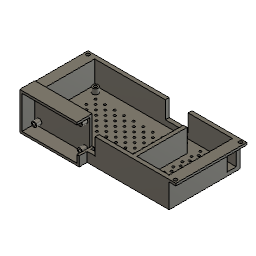
PCB+Case (Autodesk Fusion 360 design; units mm, degrees)
Autodesk Fusion 360 part; units mm, degrees
sketch "Sketch1" plane through (0, 0, 0) normal (0, 1, 0) x (1, 0, 0)
  line L0 (-72.5, 44.98) -> (120.5, 44.98)
  line L1 (120.5, 44.98) -> (120.5, -49.32)
  line L2 (120.5, -49.32) -> (-72.5, -49.32)
  line L3 (-72.5, -49.32) -> (-72.5, 44.98)
  line L4 (-67.5, 39.83) -> (67.5, 39.83)
  line L5 (67.5, 39.83) -> (67.5, -39.83)
  line L6 (67.5, -39.83) -> (-67.5, -39.83)
  line L7 (-67.5, -39.83) -> (-67.5, 39.83)
  circle A0 centre (-58.42, 31.75) radius 1.9
  circle A1 centre (-58.42, -31.75) radius 1.9
  circle A2 centre (58.42, 31.75) radius 1.9
  circle A3 centre (58.42, -31.75) radius 1.9
  circle A4 centre (-58.42, 31.75) radius 3.9
  circle A5 centre (58.42, 31.75) radius 3.9
  circle A6 centre (58.42, -31.75) radius 3.9
  circle A7 centre (-58.42, -31.75) radius 3.9
  line L8 (72.5, 39.83) -> (115.5, 39.83)
  line L9 (115.5, 39.83) -> (115.5, -44.17)
  line L10 (115.5, -44.17) -> (72.5, -44.17)
  line L11 (72.5, -44.17) -> (72.5, 39.83)
  line L12 (67.5, 39.83) -> (72.5, 39.83) construction
  dimension "d1" = 135
  dimension "d2" = 67.5
  dimension "d3" = 79.66
  dimension "d4" = 39.83
  dimension "d5" = 5.15
  dimension "d8" = 5
  dimension "d9" = 58.42
  dimension "d10" = 58.42
  dimension "d11" = 58.42
  dimension "d12" = 58.42
  dimension "d13" = 31.75
  dimension "d14" = 31.75
  dimension "d15" = 31.75
  dimension "d16" = 31.75
  dimension "d17" = 3.8
  dimension "d18" = 3.8
  dimension "d19" = 3.8
  dimension "d20" = 3.8
  dimension "d21" = 7.8
  dimension "d22" = 7.8
  dimension "d23" = 7.8
  dimension "d24" = 7.8
  dimension "d111" = 43
  dimension "d112" = 84
  dimension "d113" = 5.15
  dimension "d114" = 5
  dimension "d115" = 5
  constraint horizontal L0
  constraint vertical L1
  constraint horizontal L2
  constraint vertical L3
  constraint horizontal L4
  constraint vertical L5
  constraint horizontal L6
  constraint vertical L7
  constraint concentric A0 A4
  constraint concentric A2 A5
  constraint concentric A3 A6
  constraint concentric A1 A7
  constraint horizontal L8
  constraint vertical L9
  constraint horizontal L10
  constraint vertical L11
  constraint horizontal L12
  measures "d1" distance of L4.start L4.end
  measures "d2" distance of origin L5
  measures "d3" distance of L4.start L6.end
  measures "d4" distance of origin L4
  measures "d5" distance of L0 L4
  measures "d8" distance of L3 L7
  measures "d9" horizontal distance of origin A0.centre
  measures "d10" horizontal distance of origin A2.centre
  measures "d11" horizontal distance of origin A1.centre
  measures "d12" horizontal distance of origin A3.centre
  measures "d13" vertical distance of origin A0.centre
  measures "d14" vertical distance of origin A2.centre
  measures "d15" vertical distance of origin A1.centre
  measures "d16" vertical distance of origin A3.centre
  measures "d17" diameter of A0
  measures "d18" diameter of A2
  measures "d19" diameter of A1
  measures "d20" diameter of A3
  measures "d21" diameter of A4
  measures "d22" diameter of A5
  measures "d23" diameter of A7
  measures "d24" diameter of A6
  measures "d111" distance of L8.start L8.end
  measures "d112" distance of L8.end L9.end
  measures "d113" distance of L2 L10
  measures "d114" distance of L1 L9
  measures "d115" distance of L5 L11
extrude "Extrude1" add sketch "Sketch1" along normal blind 5 contours L4 L5 L6 L7 | A4 | A5 | A6 | A7 | L8 L9 L10 L11 makes body 1 at (-18.887, 0, 10.2448) makes body 2 at (86.8333, 0, 16.17)
extrude "Extrude3" add sketch "Sketch1" along normal blind 35 contours L0 L1 L2 L3 bodies 1 2
extrude "Extrude15" add sketch "Sketch1" along normal blind 5 contours A0 | A1 | A2 | A3 bodies 1
extrude "Extrude16" add sketch "Sketch1" along normal blind 12 contours A4 | A5 | A6 | A7 bodies 1
sketch "Sketch11" plane through (0, 35, 0) normal (0, 1, 0) x (-1, 0, 0)
  line L0 (-67.5, 39.83) -> (67.5, 39.83)
  line L1 (67.5, 39.83) -> (67.5, -39.83)
  line L2 (67.5, -39.83) -> (-67.5, -39.83)
  line L3 (-67.5, -39.83) -> (-67.5, 39.83)
  line L4 (-115.5, 44.17) -> (-72.5, 44.17)
  line L5 (-72.5, 44.17) -> (-72.5, -39.83)
  line L6 (-72.5, -39.83) -> (-115.5, -39.83)
  line L7 (-115.5, -39.83) -> (-115.5, 44.17)
  line L8 (72.5, 49.32) -> (-120.5, 49.32)
  line L9 (-120.5, 49.32) -> (-120.5, -44.98)
  line L10 (-120.5, -44.98) -> (72.5, -44.98)
  line L11 (72.5, -44.98) -> (72.5, 49.32)
  line L12 (72.5, 49.32) -> (-67.5, 49.32)
  line L13 (-67.5, 49.32) -> (-67.5, 44.83)
  line L14 (-67.5, 44.83) -> (72.5, 44.83)
  line L15 (72.5, 44.83) -> (72.5, 49.32)
  line L16 (-67.5, 44.83) -> (-67.5, 39.83)
  dimension "d117" = 5
  constraint horizontal L12
  constraint vertical L13
  constraint horizontal L14
  constraint vertical L15
  constraint coincident L8.start L11.end
  constraint coincident L0.start L3.end
  constraint vertical L16
  measures "d117" distance of L0 L14
extrude "Extrude11" cut sketch "Sketch11" against normal up to surface (35 mm away) contours L8 L11 L12 L13 L14 L15 bodies 1
sketch "Sketch2" plane through (0, 35, 0) normal (0, 1, 0) x (-1, 0, 0)
  line L0 (-67.5, 39.83) -> (67.5, 39.83)
  line L1 (67.5, 39.83) -> (67.5, -39.83)
  line L2 (67.5, -39.83) -> (-67.5, -39.83)
  line L3 (-67.5, -39.83) -> (-67.5, 39.83)
  line L4 (-67.5, 49.32) -> (-120.5, 49.32)
  line L5 (-120.5, 49.32) -> (-120.5, -44.98)
  line L6 (-120.5, -44.98) -> (72.5, -44.98)
  line L7 (72.5, -44.98) -> (72.5, 44.83)
  line L8 (81.5, -44.98) -> (-129.5, -44.98)
  line L9 (-129.5, -44.98) -> (-129.5, 49.32)
  line L10 (81.5, 44.83) -> (81.5, -44.98)
  circle A0 centre (77, 40.33) radius 2.25
  circle A1 centre (77, -40.48) radius 2.25
  circle A2 centre (-125, -40.98) radius 2.25
  circle A3 centre (-125, 45.32) radius 2.25
  line L11 (-115.5, 44.17) -> (-72.5, 44.17)
  line L12 (-72.5, 44.17) -> (-72.5, -39.83)
  line L13 (-72.5, -39.83) -> (-115.5, -39.83)
  line L14 (-115.5, -39.83) -> (-115.5, 44.17)
  line L15 (-67.5, 44.83) -> (-67.5, 49.32)
  line L16 (72.5, 44.83) -> (-67.5, 44.83)
  line L17 (-129.5, 49.32) -> (-120.5, 49.32)
  line L18 (72.5, 44.83) -> (81.5, 44.83)
  point P0 (-24, -44.98)
  dimension "d33" = 9
  dimension "d39" = 4.5
  dimension "d40" = 4.5
  dimension "d41" = 4.5
  dimension "d42" = 4.5
  dimension "d43" = 4
  dimension "d44" = 4.5
  dimension "d46" = 4.5
  dimension "d47" = 4.5
  dimension "d48" = 4.5
  dimension "d50" = 4.5
  dimension "d116" = 9
  dimension "d121" = 4
  dimension "d122" = 4.5
  constraint horizontal L8
  constraint vertical L9
  constraint vertical L10
  constraint midpoint L6 P0
  constraint coincident L8 P0
  constraint coincident L4.end L5.start
  constraint perpendicular L5 L17
  constraint coincident L7.end L16.start
  constraint horizontal L18
  measures "d33" distance of L7 L10
  measures "d39" distance of L10 A1.centre
  measures "d40" distance of L8 A1.centre
  measures "d41" diameter of A1
  measures "d42" distance of L9 A2.centre
  measures "d43" distance of L8 A2.centre
  measures "d44" diameter of A2
  measures "d46" distance of L10 A0.centre
  measures "d47" diameter of A0
  measures "d48" distance of L9 A3.centre
  measures "d50" diameter of A3
  measures "d116" distance of L5 L9
  measures "d121" distance of A3.centre L17
  measures "d122" distance of A0.centre L18
extrude "Extrude4" add sketch "Sketch2" against normal blind 3 contours L5 L8 L9 L17 | L7 L8 L10 L18 bodies 1
sketch "Sketch7" plane through (0, 35, 0) normal (0, 1, 0) x (-1, 0, 0)
  line L0 (81.5, -44.98) -> (81.5, 44.83)
  line L1 (-67.5, 49.32) -> (-129.5, 49.32)
  circle A0 centre (77, 40.33) radius 2.25
  line L2 (67.5, 39.83) -> (-11.62, 39.83)
  line L3 (67.5, 59.83) -> (67.5, 39.83)
  line L4 (-11.62, 39.83) -> (-11.62, 59.83)
  line L5 (67.5, 59.83) -> (-11.62, 59.83)
  line L6 (-129.5, -44.98) -> (81.5, -44.98)
  circle A1 centre (77, -40.48) radius 2.25
  line L7 (-67.5, -39.83) -> (-67.5, 39.83)
  line L8 (-67.5, 39.83) -> (67.5, 39.83)
  line L9 (67.5, 39.83) -> (67.5, -39.83)
  line L10 (67.5, -39.83) -> (-67.5, -39.83)
  line L11 (81.5, 44.83) -> (-67.5, 44.83)
  line L12 (-67.5, 44.83) -> (-67.5, 49.32)
  line L13 (-129.5, 49.32) -> (-129.5, -44.98)
  circle A2 centre (-125, 45.32) radius 2.25
  circle A3 centre (-125, -40.98) radius 2.25
  line L14 (-115.5, 44.17) -> (-72.5, 44.17)
  line L15 (-72.5, 44.17) -> (-72.5, -39.83)
  line L16 (-72.5, -39.83) -> (-115.5, -39.83)
  line L17 (-115.5, -39.83) -> (-115.5, 44.17)
  dimension "d59" = 20
  dimension "d60" = 79.12
  constraint horizontal L2
  constraint vertical L3
  constraint perpendicular L3 L5
  constraint coincident L2 L3.end
  constraint coincident L3 L2.start
  constraint perpendicular L4 L5
  measures "d59" distance of L2.start L3.start
  measures "d60" distance of L2.start L2.end
extrude "Extrude6" add sketch "Sketch7" against normal up to surface (35 mm away) contours L3 L4 L5 L11 bodies 1
extrude "Extrude7" add sketch "Sketch7" along normal blind 14.91 contours L3 L4 L5 L11 | L2 L3 L4 L8 L11 bodies 1
sketch "Sketch8" plane through (0, 0, 59.83) normal (0, 0, 1) x (1, 0, 0)
  line L0 (11.62, 0) -> (11.62, 49.91)
  line L1 (11.62, 49.91) -> (-67.5, 49.91)
  line L2 (-67.5, 49.91) -> (-67.5, 0)
  line L3 (-64.5, 46.91) -> (8.62, 46.91)
  line L4 (8.62, 46.91) -> (8.62, 3)
  line L5 (8.62, 3) -> (-64.5, 3)
  line L6 (-64.5, 3) -> (-64.5, 46.91)
  line L7 (-67.5, 0) -> (11.62, 0)
  dimension "d65" = 3
  dimension "d66" = 3
  dimension "d67" = 3
  dimension "d140" = 3
  constraint horizontal L3
  constraint vertical L4
  constraint horizontal L5
  constraint vertical L6
  measures "d65" distance of L2 L6
  measures "d66" distance of L1 L3
  measures "d67" distance of L0 L4
  measures "d140" distance of L5 L7
extrude "Extrude8" cut sketch "Sketch8" against normal blind 17 contours L3 L4 L5 L6 bodies 1
sketch "Sketch9" plane through (0, 0, 42.83) normal (0, 0, 1) x (1, 0, 0)
  line L0 (-64.5, 3) -> (8.62, 3)
  line L1 (8.62, 3) -> (8.62, 46.91)
  line L2 (-64.5, 46.91) -> (-64.5, 3)
  circle A0 centre (-58.42, 40.83) radius 1.9
  circle A1 centre (2.54, 40.83) radius 1.9
  circle A2 centre (-58.42, 9.08) radius 1.9
  circle A3 centre (2.54, 9.08) radius 1.9
  line L3 (-64.5, 24.955) -> (8.62, 24.955) construction
  line L4 (8.62, 46.91) -> (-64.5, 46.91)
  circle A4 centre (-58.42, 9.08) radius 3.4
  circle A5 centre (-58.42, 40.83) radius 3.4
  circle A6 centre (2.54, 40.83) radius 3.4
  circle A7 centre (2.54, 9.08) radius 3.4
  line L5 (-13.97, 31.94) -> (-62.23, 31.94)
  line L6 (-62.23, 31.94) -> (-62.23, 37.02)
  line L7 (-62.23, 37.02) -> (-26.67, 37.02)
  line L8 (-26.67, 37.02) -> (-26.67, 43.37)
  line L9 (-26.67, 43.37) -> (-13.97, 43.37)
  line L10 (-13.97, 43.37) -> (-13.97, 31.94)
  dimension "d79" = 3.8
  dimension "d80" = 3.8
  dimension "d81" = 3.8
  dimension "d82" = 3.8
  dimension "d85" = 6.08
  dimension "d86" = 6.08
  dimension "d87" = 6.08
  dimension "d88" = 6.08
  dimension "d89" = 6.08
  dimension "d91" = 6.08
  dimension "d131" = 6.08
  dimension "d132" = 6.08
  dimension "d133" = 6.8
  dimension "d134" = 6.8
  dimension "d135" = 6.8
  dimension "d136" = 6.8
  dimension "d138" = 22.86
  dimension "d141" = 5.08
  dimension "d142" = 3.81
  dimension "d143" = 31.75
  dimension "d144" = 12.7
  dimension "d145" = 2.54
  constraint midpoint L2 L3.start
  constraint midpoint L1 L3.end
  constraint concentric A2 A4
  constraint concentric A0 A5
  constraint concentric A1 A6
  constraint concentric A3 A7
  constraint horizontal L5
  constraint vertical L6
  constraint perpendicular L6 L7
  constraint perpendicular L7 L8
  constraint perpendicular L8 L9
  constraint perpendicular L9 L10
  measures "d79" diameter of A2
  measures "d80" diameter of A0
  measures "d81" diameter of A1
  measures "d82" diameter of A3
  measures "d85" distance of L0 A2.centre
  measures "d86" distance of L2 A2.centre
  measures "d87" distance of L0 A3.centre
  measures "d88" distance of L1 A3.centre
  measures "d89" distance of L2 A0.centre
  measures "d91" distance of L1 A1.centre
  measures "d131" distance of A0.centre L4
  measures "d132" distance of A1.centre L4
  measures "d133" diameter of A4
  measures "d134" diameter of A5
  measures "d135" diameter of A6
  measures "d136" diameter of A7
  measures "d138" distance of A2.centre L5
  measures "d141" distance of L6.end L5.end
  measures "d142" distance of A0.centre L6
  measures "d143" distance of A0.centre L8
  measures "d144" distance of L8.end L9.end
  measures "d145" distance of A0.centre L9
extrude "Extrude9" add sketch "Sketch9" along normal blind 7 contours A4 | A5 | A6 | A7 bodies 1
extrude "Extrude14" cut sketch "Sketch9" against normal up to surface (3 mm away) contours L5 L6 L7 L8 L9 L10 bodies 1
sketch "Sketch5" plane through (0, 0, -44.98) normal (0, 0, -1) x (-1, 0, 0)
  line L0 (72.5, 32) -> (81.5, 32)
  line L1 (-120.5, 32) -> (-120.5, 0)
  line L2 (-120.5, 0) -> (72.5, 0)
  line L3 (72.5, 0) -> (72.5, 32)
  line L4 (81.5, 35) -> (-129.5, 35)
  line L5 (72.5, 32) -> (81.5, 32)
  line L6 (81.5, 32) -> (81.5, 35)
  line L7 (81.5, 32) -> (81.5, 35)
  line L8 (81.5, 35) -> (-129.5, 35)
  line L9 (-120.5, 0) -> (72.5, 0)
  line L10 (72.5, 0) -> (72.5, 32)
  line L11 (-120.5, 32) -> (-120.5, 0)
  line L12 (-56.52, 12) -> (-26.52, 12)
  line L13 (-26.52, 12) -> (-26.52, 35)
  line L14 (-26.52, 35) -> (-56.52, 35)
  line L15 (-56.52, 35) -> (-56.52, 12)
  line L16 (-56.52, 5) -> (-56.52, 35) construction
  line L17 (-129.5, 35) -> (-129.5, 32)
  line L18 (-129.5, 32) -> (-120.5, 32)
  line L19 (-129.5, 35) -> (-129.5, 32)
  line L20 (-129.5, 32) -> (-120.5, 32)
  line L21 (-72.5, 5) -> (-115.5, 5)
  line L22 (-115.5, 5) -> (-72.5, 5)
  line L23 (-60.32, 12) -> (-56.52, 12)
  line L24 (-54.52, 12) -> (-62.32, 12)
  dimension "d95" = 30
  constraint horizontal L12
  constraint vertical L13
  constraint horizontal L14
  constraint vertical L15
  constraint coincident L8 L13.end
  constraint coincident L4 L14.end
  constraint perpendicular L4 L16
  constraint coincident L12.start L16
  constraint coincident L12 L24.start
  constraint coincident L15 L12.start
  measures "d95" distance of L13.end L14.end
extrude "Extrude5" cut sketch "Sketch5" along normal up to surface (0 mm away) and the other way up to surface (5.15 mm away) contours L4 L8 L12 L13 L14 L15 L24 bodies 1
sketch "Sketch10" plane through (0, 0, 49.32) normal (0, 0, 1) x (1, 0, 0)
  line L0 (129.5, 35) -> (67.5, 35)
  line L1 (8.62, 3) -> (8.62, 46.91)
  line L2 (8.62, 46.91) -> (8.62, 3)
  line L3 (22.23, 49.91) -> (8.62, 49.91)
  line L4 (8.62, 49.91) -> (8.62, 12.874)
  line L5 (8.62, 12.874) -> (22.23, 12.874)
  line L6 (11.62, 49.91) -> (-67.5, 49.91)
  line L7 (11.62, 49.91) -> (24.4054, 49.91) construction
  line L8 (22.23, 49.91) -> (22.23, 12.874)
  line L9 (67.5, 0) -> (120.5, 0)
  line L10 (120.5, 0) -> (120.5, 32)
  line L11 (120.5, 32) -> (129.5, 32)
  line L12 (-67.5, 49.91) -> (11.62, 49.91)
  line L13 (67.5, 35) -> (67.5, 0)
  line L14 (129.5, 32) -> (129.5, 35)
  line L15 (72.5, 5) -> (115.5, 5)
  line L16 (115.5, 5) -> (72.5, 5)
  constraint horizontal L3
  constraint vertical L4
  constraint horizontal L5
  constraint coincident L2 L4.end
  constraint coincident L6.start L7.start
  constraint parallel L6 L7
  constraint coincident L3.start L7
  constraint perpendicular L3 L8
extrude "Extrude10" cut sketch "Sketch10" along normal up to surface (-9.49 mm away) and the other way up to surface (-10.51 mm away) contours L1 L2 L3 L4 L5 L6 L8 L12 bodies 1
sketch "Sketch12" plane through (120.5, 0, 0) normal (1, 0, 0) x (0, 0, -1)
  line L0 (44.98, 32) -> (-49.32, 32)
  line L1 (-44.17, 5) -> (39.83, 5)
  line L2 (39.83, 5) -> (-44.17, 5)
  line L3 (-49.32, 32) -> (44.98, 32)
  line L4 (43.23, 32) -> (38.73, 32)
  line L5 (-43.07, 32) -> (-47.57, 32)
  line L6 (39.83, 5) -> (27.83, 5)
  line L7 (27.83, 5) -> (27.83, 25)
  line L8 (27.83, 25) -> (39.83, 25)
  line L9 (39.83, 25) -> (39.83, 5)
  line L10 (-49.32, 32) -> (-49.32, 0)
  line L11 (-49.32, 0) -> (44.98, 0)
  line L12 (44.98, 0) -> (44.98, 32)
  line L13 (44.98, 32) -> (-49.32, 32)
  dimension "d123" = 12
  dimension "d158" = 20
  constraint horizontal L6
  constraint vertical L7
  constraint horizontal L8
  constraint vertical L9
  constraint coincident L1.end L2.start
  measures "d123" distance of L1.end L6.end
  measures "d158" distance of L1.end L8.end
extrude "Extrude12" cut sketch "Sketch12" against normal up to surface (5 mm away) contours L1 L2 L6 L7 L8 L9 bodies 1
sketch "Sketch14" plane through (0, 0, 0) normal (0, -1, 0) x (1, 0, 0)
  line L0 (67.5, 44.83) -> (11.62, 44.83)
  line L1 (11.62, 44.83) -> (11.62, 59.83)
  line L2 (11.62, 59.83) -> (-67.5, 59.83)
  line L3 (-67.5, 59.83) -> (-67.5, 44.83)
  line L4 (-67.5, 44.83) -> (-72.5, 44.83)
  line L5 (-72.5, 44.83) -> (-72.5, -44.98)
  line L6 (-72.5, -44.98) -> (120.5, -44.98)
  line L7 (120.5, -44.98) -> (120.5, 49.32)
  line L8 (120.5, 49.32) -> (67.5, 49.32)
  line L9 (67.5, 49.32) -> (67.5, 44.83)
  line L10 (11.62, 44.83) -> (67.5, 44.83)
  line L11 (67.5, 44.83) -> (67.5, 49.32)
  line L12 (67.5, 49.32) -> (11.62, 49.32)
  line L13 (11.62, 49.32) -> (11.62, 44.83)
  line L14 (22.23, 44.83) -> (22.23, 49.32)
  point P0 (22.23, 44.83)
  constraint horizontal L10
  constraint vertical L11
  constraint horizontal L12
  constraint vertical L13
  constraint coincident L8.end L9.start
  constraint coincident L0.end L1.start
  constraint coincident P0 L14.start
  constraint coincident L12 L14.end
  constraint perpendicular L12 L14
extrude "Extrude17" add sketch "Sketch14" against normal up to surface (35 mm away) contours L0 L9 L10 L11 L12 L14 bodies 1
extrude "Extrude19" add sketch "Sketch14" against normal up to surface (12.874 mm away) contours L0 L1 L10 L12 L13 L14 bodies 1
sketch "Sketch15" plane through (0, 35, 0) normal (0, 1, 0) x (-1, 0, 0)
  line L0 (-115.5, 44.17) -> (-72.5, 44.17)
  line L1 (-72.5, 44.17) -> (-72.5, -39.83)
  line L2 (-72.5, -39.83) -> (-115.5, -39.83)
  line L3 (-115.5, -39.83) -> (-115.5, 44.17)
  circle A0 centre (-125, -40.98) radius 2.25
  circle A1 centre (-125, 45.32) radius 2.25
  line L4 (-22.23, 39.83) -> (-22.23, 49.32)
  line L5 (-22.23, 49.32) -> (-129.5, 49.32)
  line L6 (-129.5, 49.32) -> (-129.5, -44.98)
  line L7 (-129.5, -44.98) -> (-56.52, -44.98)
  line L8 (-56.52, -44.98) -> (-56.52, -39.83)
  line L9 (-56.52, -39.83) -> (-67.5, -39.83)
  line L10 (-67.5, -39.83) -> (-67.5, 39.83)
  line L11 (-67.5, 39.83) -> (-22.23, 39.83)
  line L12 (-11.62, 44.17) -> (-67.5, 44.17)
  line L13 (-67.5, 44.17) -> (-67.5, 39.83)
  line L14 (-67.5, 39.83) -> (-11.62, 39.83)
  line L15 (-11.62, 39.83) -> (-11.62, 44.17)
  line L16 (-72.5, 44.17) -> (-67.5, 44.17)
  line L17 (-22.23, 49.32) -> (-22.23, 39.83) construction
  line L18 (-22.23, 39.83) -> (-8.62, 39.83) construction
  line L19 (-8.62, 39.83) -> (-8.62, 42.83) construction
  line L20 (-8.62, 42.83) -> (-8.62, 59.83) construction
  line L21 (-8.62, 59.83) -> (-11.62, 59.83) construction
  line L22 (-11.62, 59.83) -> (-11.62, 49.32) construction
  line L23 (-11.62, 49.32) -> (-22.23, 49.32) construction
  line L24 (-11.62, 44.17) -> (-11.62, 49.32) construction
  constraint horizontal L12
  constraint vertical L13
  constraint horizontal L14
  constraint vertical L15
  constraint coincident L10.end L11.start
  constraint coincident L0.end L1.start
  constraint horizontal L16
  constraint coincident L22.end L23.start
  constraint vertical L24
extrude "Extrude18" cut sketch "Sketch15" against normal up to surface (30 mm away) contours L4 L11 L12 L13 L14 | L4 L12 L14 L15 bodies 1
sketch "Sketch16" plane through (67.5, 0, 0) normal (-1, 0, 0) x (0, 0, 1)
  line L0 (-39.83, 5) -> (44.17, 5)
  line L1 (44.17, 5) -> (44.17, 35)
  line L2 (44.17, 35) -> (-39.83, 35)
  line L3 (-39.83, 35) -> (-39.83, 5)
  line L4 (-39.83, 35) -> (-22.83, 35)
  line L5 (-22.83, 35) -> (-22.83, 5)
  line L6 (-22.83, 5) -> (-39.83, 5)
  line L7 (-39.83, 5) -> (-39.83, 35)
  line L8 (-39.83, 25) -> (-27.83, 25)
  dimension "d188" = 5
  constraint horizontal L4
  constraint vertical L5
  constraint horizontal L6
  constraint vertical L7
  constraint coincident L0 L5.end
  constraint coincident L2.end L3.start
  measures "d188" distance of L5 L8.end
extrude "Extrude20" cut sketch "Sketch16" against normal up to surface (5 mm away) contours L0 L2 L3 L4 L5 L6 L7 bodies 1
sketch "Sketch17" plane through (0, 5, 0) normal (0, 1, 0) x (-1, 0, 0)
  circle A0 centre (58.42, -31.75) radius 3.9
  circle A1 centre (58.42, 31.75) radius 3.9
  line L0 (67.5, 39.83) -> (-11.62, 39.83)
  line L1 (-11.62, 39.83) -> (-11.62, 44.17)
  line L2 (-11.62, 44.17) -> (-67.5, 44.17)
  line L3 (-120.5, -39.83) -> (67.5, -39.83)
  line L4 (67.5, -39.83) -> (67.5, 39.83)
  circle A2 centre (-58.42, 31.75) radius 3.9
  circle A3 centre (-58.42, -31.75) radius 3.9
  line L5 (-58.42, 31.75) -> (-58.42, -31.75) construction
  line L6 (-58.42, -31.75) -> (58.42, -31.75) construction
  line L7 (58.42, -31.75) -> (58.42, 31.75) construction
  line L8 (58.42, 31.75) -> (-58.42, 31.75) construction
  circle A4 centre (0, 0) radius 1.5
  line L9 (-58.42, 0) -> (58.42, 0) construction
  line L10 (0, -31.75) -> (0, 31.75) construction
  circle A5 centre (-50.8, -24.13) radius 1.5
  circle A6 centre (-38.1, -24.13) radius 1.5
  circle A7 centre (-25.4, -24.13) radius 1.5
  circle A8 centre (-12.7, -24.13) radius 1.5
  circle A9 centre (0, -24.13) radius 1.5
  circle A10 centre (12.7, -24.13) radius 1.5
  circle A11 centre (25.4, -24.13) radius 1.5
  circle A12 centre (38.1, -24.13) radius 1.5
  circle A13 centre (50.8, -24.13) radius 1.5
  circle A14 centre (-50.8, -12.065) radius 1.5
  circle A15 centre (-38.1, -12.065) radius 1.5
  circle A16 centre (-25.4, -12.065) radius 1.5
  circle A17 centre (-12.7, -12.065) radius 1.5
  circle A18 centre (0, -12.065) radius 1.5
  circle A19 centre (12.7, -12.065) radius 1.5
  circle A20 centre (25.4, -12.065) radius 1.5
  circle A21 centre (38.1, -12.065) radius 1.5
  circle A22 centre (50.8, -12.065) radius 1.5
  circle A23 centre (-50.8, 0) radius 1.5
  circle A24 centre (-38.1, 0) radius 1.5
  circle A25 centre (-25.4, 0) radius 1.5
  circle A26 centre (-12.7, 0) radius 1.5
  circle A27 centre (12.7, 0) radius 1.5
  circle A28 centre (25.4, 0) radius 1.5
  circle A29 centre (38.1, 0) radius 1.5
  circle A30 centre (50.8, 0) radius 1.5
  circle A31 centre (-50.8, 12.065) radius 1.5
  circle A32 centre (-38.1, 12.065) radius 1.5
  circle A33 centre (-25.4, 12.065) radius 1.5
  circle A34 centre (-12.7, 12.065) radius 1.5
  circle A35 centre (0, 12.065) radius 1.5
  circle A36 centre (12.7, 12.065) radius 1.5
  circle A37 centre (25.4, 12.065) radius 1.5
  circle A38 centre (38.1, 12.065) radius 1.5
  circle A39 centre (50.8, 12.065) radius 1.5
  circle A40 centre (-50.8, 24.13) radius 1.5
  circle A41 centre (-38.1, 24.13) radius 1.5
  circle A42 centre (-25.4, 24.13) radius 1.5
  circle A43 centre (-12.7, 24.13) radius 1.5
  circle A44 centre (0, 24.13) radius 1.5
  circle A45 centre (12.7, 24.13) radius 1.5
  circle A46 centre (25.4, 24.13) radius 1.5
  circle A47 centre (38.1, 24.13) radius 1.5
  circle A48 centre (50.8, 24.13) radius 1.5
  line L11 (50.8, -24.13) -> (50.8, -12.065) construction
  line L12 (50.8, -12.065) -> (38.1, -12.065) construction
  line L13 (38.1, -12.065) -> (38.1, -24.13) construction
  line L14 (38.1, -24.13) -> (50.8, -24.13) construction
  line L15 (50.8, -18.0975) -> (38.1, -18.0975) construction
  line L16 (44.45, -24.13) -> (44.45, -12.065) construction
  circle A49 centre (44.45, -18.0975) radius 1.5
  circle A50 centre (31.75, -18.0975) radius 1.5
  circle A51 centre (19.05, -18.0975) radius 1.5
  circle A52 centre (6.35, -18.0975) radius 1.5
  circle A53 centre (-6.35, -18.0975) radius 1.5
  circle A54 centre (-19.05, -18.0975) radius 1.5
  circle A55 centre (-31.75, -18.0975) radius 1.5
  circle A56 centre (-44.45, -18.0975) radius 1.5
  circle A57 centre (44.45, -6.0325) radius 1.5
  circle A58 centre (31.75, -6.0325) radius 1.5
  circle A59 centre (19.05, -6.0325) radius 1.5
  circle A60 centre (6.35, -6.0325) radius 1.5
  circle A61 centre (-6.35, -6.0325) radius 1.5
  circle A62 centre (-19.05, -6.0325) radius 1.5
  circle A63 centre (-31.75, -6.0325) radius 1.5
  circle A64 centre (-44.45, -6.0325) radius 1.5
  circle A65 centre (44.45, 6.0325) radius 1.5
  circle A66 centre (31.75, 6.0325) radius 1.5
  circle A67 centre (19.05, 6.0325) radius 1.5
  circle A68 centre (6.35, 6.0325) radius 1.5
  circle A69 centre (-6.35, 6.0325) radius 1.5
  circle A70 centre (-19.05, 6.0325) radius 1.5
  circle A71 centre (-31.75, 6.0325) radius 1.5
  circle A72 centre (-44.45, 6.0325) radius 1.5
  circle A73 centre (44.45, 18.0975) radius 1.5
  circle A74 centre (31.75, 18.0975) radius 1.5
  circle A75 centre (19.05, 18.0975) radius 1.5
  circle A76 centre (6.35, 18.0975) radius 1.5
  circle A77 centre (-6.35, 18.0975) radius 1.5
  circle A78 centre (-19.05, 18.0975) radius 1.5
  circle A79 centre (-31.75, 18.0975) radius 1.5
  circle A80 centre (-44.45, 18.0975) radius 1.5
  line L17 (-115.5, 44.17) -> (-115.5, -27.83)
  line L18 (-115.5, -27.83) -> (-120.5, -27.83)
  line L19 (-120.5, -27.83) -> (-120.5, -39.83)
  line L20 (-67.5, 44.17) -> (-67.5, -22.83)
  line L21 (-67.5, -22.83) -> (-72.5, -22.83)
  line L22 (-72.5, -22.83) -> (-72.5, 44.17)
  line L23 (-72.5, 44.17) -> (-115.5, 44.17)
  dimension "d166" = 50.8
  dimension "d167" = 24.13
  dimension "d168" = 3
  dimension "d171" = 3
  dimension "d174" = -88.9
  dimension "d175" = 36.195
  constraint coincident A2.centre L5.start
  constraint coincident A3.centre L5.end
  constraint coincident A0.centre L6.end
  constraint coincident A1.centre L7.end
  constraint coincident A4.centre origin
  constraint midpoint L5 L9.start
  constraint midpoint L7 L9.end
  constraint midpoint L6 L10.start
  constraint midpoint L8 L10.end
  constraint midpoint L11 L15.start
  constraint midpoint L13 L15.end
  constraint midpoint L14 L16.start
  constraint midpoint L12 L16.end
  constraint midpoint L15 A49.centre
  constraint perpendicular L11 L14
  constraint perpendicular L12 L13
  constraint perpendicular L13 L14
  constraint coincident A22.centre L12
  constraint coincident A22.centre L11
  constraint coincident A12.centre L13
  constraint coincident A12.centre L14
  constraint coincident A13.centre L11.start
  measures "d168" diameter of A4
  measures "d171" diameter of A49
extrude "Extrude21" cut sketch "Sketch17" against normal up to surface (5 mm away) contours A4 | A5 | A6 | A7 | A8 | A9 | A10 | A11 | A12 | A13 | A14 | A15 | A16 | A17 | A18 | A19 | A20 | A21 | A22 | A23 | A24 | A25 | A26 | A27 | A28 | A29 | A30 | A31 | A32 | A33 | A34 | A35 | A36 | A37 | A38 | A39 | A40 | A41 | A42 | A43 | A44 | A45 | A46 | A47 | A48 | A49 | A50 | A51 | A52 | A53 | A54 | A55 | A56 | A57 | A58 | A59 | A60 | A61 | A62 | A63 | A64 | A65 | A66 | A67 | A68 | A69 | A70 | A71 | A72 | A73 | A74 | A75 | A76 | A77 | A78 | A79 | A80 bodies 1
sketch "Sketch18" plane through (0, 5, 0) normal (0, 1, 0) x (-1, 0, 0)
  line L0 (-11.62, 44.17) -> (-67.5, 44.17)
  line L1 (-115.5, 44.17) -> (-115.5, -27.83)
  line L2 (-115.5, -27.83) -> (-120.5, -27.83)
  line L3 (-120.5, -27.83) -> (-120.5, -39.83)
  line L4 (-120.5, -39.83) -> (67.5, -39.83)
  circle A0 centre (-31.75, 6.0325) radius 1.5
  circle A1 centre (-31.75, -18.0975) radius 1.5
  circle A2 centre (-6.35, -18.0975) radius 1.5
  circle A3 centre (-6.35, 18.0975) radius 1.5
  circle A4 centre (19.05, 18.0975) radius 1.5
  circle A5 centre (6.35, -18.0975) radius 1.5
  circle A6 centre (31.75, 6.0325) radius 1.5
  circle A7 centre (44.45, -6.0325) radius 1.5
  circle A8 centre (38.1, 24.13) radius 1.5
  circle A9 centre (0, 24.13) radius 1.5
  circle A10 centre (-25.4, -24.13) radius 1.5
  circle A11 centre (-12.7, -24.13) radius 1.5
  circle A12 centre (12.7, 12.065) radius 1.5
  circle A13 centre (50.8, -24.13) radius 1.5
  circle A14 centre (-50.8, -24.13) radius 1.5
  circle A15 centre (12.7, -12.065) radius 1.5
  circle A16 centre (-25.4, -12.065) radius 1.5
  circle A17 centre (50.8, 12.065) radius 1.5
  circle A18 centre (-38.1, 0) radius 1.5
  circle A19 centre (-50.8, 24.13) radius 1.5
  circle A20 centre (-12.7, -12.065) radius 1.5
  circle A21 centre (-38.1, -12.065) radius 1.5
  circle A22 centre (-38.1, -24.13) radius 1.5
  circle A23 centre (25.4, 0) radius 1.5
  circle A24 centre (25.4, -24.13) radius 1.5
  circle A25 centre (12.7, -24.13) radius 1.5
  circle A26 centre (38.1, -12.065) radius 1.5
  circle A27 centre (-38.1, 24.13) radius 1.5
  circle A28 centre (0, 12.065) radius 1.5
  circle A29 centre (-25.4, 0) radius 1.5
  circle A30 centre (44.45, -18.0975) radius 1.5
  circle A31 centre (31.75, 18.0975) radius 1.5
  circle A32 centre (19.05, -18.0975) radius 1.5
  circle A33 centre (19.05, 6.0325) radius 1.5
  circle A34 centre (-6.35, 6.0325) radius 1.5
  circle A35 centre (-6.35, -6.0325) radius 1.5
  circle A36 centre (-31.75, -6.0325) radius 1.5
  circle A37 centre (-44.45, 6.0325) radius 1.5
  circle A38 centre (-31.75, 18.0975) radius 1.5
  circle A39 centre (-44.45, -18.0975) radius 1.5
  circle A40 centre (-19.05, -18.0975) radius 1.5
  circle A41 centre (-19.05, 18.0975) radius 1.5
  circle A42 centre (6.35, 18.0975) radius 1.5
  circle A43 centre (6.35, -6.0325) radius 1.5
  circle A44 centre (31.75, -6.0325) radius 1.5
  circle A45 centre (44.45, 6.0325) radius 1.5
  circle A46 centre (25.4, 24.13) radius 1.5
  circle A47 centre (38.1, 0) radius 1.5
  circle A48 centre (-50.8, -12.065) radius 1.5
  circle A49 centre (-25.4, 24.13) radius 1.5
  circle A50 centre (-38.1, 12.065) radius 1.5
  circle A51 centre (38.1, -24.13) radius 1.5
  circle A52 centre (-50.8, 0) radius 1.5
  circle A53 centre (50.8, -12.065) radius 1.5
  circle A54 centre (38.1, 12.065) radius 1.5
  circle A55 centre (-50.8, 12.065) radius 1.5
  circle A56 centre (0, -24.13) radius 1.5
  circle A57 centre (-12.7, 0) radius 1.5
  circle A58 centre (12.7, 24.13) radius 1.5
  circle A59 centre (25.4, 12.065) radius 1.5
  circle A60 centre (-25.4, 12.065) radius 1.5
  circle A61 centre (12.7, 0) radius 1.5
  circle A62 centre (-12.7, 24.13) radius 1.5
  circle A63 centre (25.4, -12.065) radius 1.5
  circle A64 centre (0, 0) radius 1.5
  circle A65 centre (50.8, 0) radius 1.5
  circle A66 centre (50.8, 24.13) radius 1.5
  circle A67 centre (0, -12.065) radius 1.5
  circle A68 centre (-12.7, 12.065) radius 1.5
  circle A69 centre (44.45, 18.0975) radius 1.5
  circle A70 centre (31.75, -18.0975) radius 1.5
  circle A71 centre (19.05, -6.0325) radius 1.5
  circle A72 centre (6.35, 6.0325) radius 1.5
  circle A73 centre (-19.05, 6.0325) radius 1.5
  circle A74 centre (-19.05, -6.0325) radius 1.5
  circle A75 centre (-44.45, -6.0325) radius 1.5
  circle A76 centre (-44.45, 18.0975) radius 1.5
  circle A77 centre (58.42, -31.75) radius 3.9
  circle A78 centre (58.42, 31.75) radius 3.9
  line L5 (67.5, 39.83) -> (-11.62, 39.83)
  line L6 (-11.62, 39.83) -> (-11.62, 44.17)
  line L7 (67.5, -39.83) -> (67.5, 39.83)
  circle A79 centre (-58.42, 31.75) radius 3.9
  circle A80 centre (-58.42, -31.75) radius 3.9
  line L8 (-67.5, 44.17) -> (-67.5, -22.83)
  line L9 (-67.5, -22.83) -> (-72.5, -22.83)
  line L10 (-72.5, -22.83) -> (-72.5, 44.17)
  line L11 (-72.5, 44.17) -> (-115.5, 44.17)
sketch "Sketch19" plane through (0, 5, 0) normal (0, 1, 0) x (-1, 0, 0)
  line L0 (-11.62, 44.17) -> (-67.5, 44.17) construction
  line L1 (-115.5, 44.17) -> (-115.5, -27.83) construction
  line L2 (-115.5, -27.83) -> (-120.5, -27.83) construction
  line L3 (-120.5, -27.83) -> (-120.5, -39.83) construction
  line L4 (-120.5, -39.83) -> (67.5, -39.83) construction
  line L5 (-72.5, 2.17) -> (-115.5, 2.17) construction
  circle A0 centre (-94, 2.17) radius 1.5
  circle A1 centre (-109, -33.83) radius 1.5
  circle A2 centre (-101.5, -33.83) radius 1.5
  circle A3 centre (-94, -33.83) radius 1.5
  circle A4 centre (-86.5, -33.83) radius 1.5
  circle A5 centre (-79, -33.83) radius 1.5
  circle A6 centre (-109, -21.83) radius 1.5
  circle A7 centre (-101.5, -21.83) radius 1.5
  circle A8 centre (-94, -21.83) radius 1.5
  circle A9 centre (-86.5, -21.83) radius 1.5
  circle A10 centre (-79, -21.83) radius 1.5
  circle A11 centre (-109, -9.83) radius 1.5
  circle A12 centre (-101.5, -9.83) radius 1.5
  circle A13 centre (-94, -9.83) radius 1.5
  circle A14 centre (-86.5, -9.83) radius 1.5
  circle A15 centre (-79, -9.83) radius 1.5
  circle A16 centre (-109, 2.17) radius 1.5
  circle A17 centre (-101.5, 2.17) radius 1.5
  circle A18 centre (-86.5, 2.17) radius 1.5
  circle A19 centre (-79, 2.17) radius 1.5
  circle A20 centre (-109, 14.17) radius 1.5
  circle A21 centre (-101.5, 14.17) radius 1.5
  circle A22 centre (-94, 14.17) radius 1.5
  circle A23 centre (-86.5, 14.17) radius 1.5
  circle A24 centre (-79, 14.17) radius 1.5
  circle A25 centre (-109, 26.17) radius 1.5
  circle A26 centre (-101.5, 26.17) radius 1.5
  circle A27 centre (-94, 26.17) radius 1.5
  circle A28 centre (-86.5, 26.17) radius 1.5
  circle A29 centre (-79, 26.17) radius 1.5
  circle A30 centre (-109, 38.17) radius 1.5
  circle A31 centre (-101.5, 38.17) radius 1.5
  circle A32 centre (-94, 38.17) radius 1.5
  circle A33 centre (-86.5, 38.17) radius 1.5
  circle A34 centre (-79, 38.17) radius 1.5
  line L6 (-79, -33.83) -> (-79, -21.83) construction
  line L7 (-79, -21.83) -> (-86.5, -21.83) construction
  line L8 (-86.5, -21.83) -> (-86.5, -33.83) construction
  line L9 (-86.5, -33.83) -> (-79, -33.83) construction
  line L10 (-79, -27.83) -> (-86.5, -27.83) construction
  line L11 (-82.75, -33.83) -> (-82.75, -21.83) construction
  circle A35 centre (-82.75, -27.83) radius 1.5
  circle A36 centre (-90.25, -27.83) radius 1.5
  circle A37 centre (-97.75, -27.83) radius 1.5
  circle A38 centre (-105.25, -27.83) radius 1.5
  circle A39 centre (-82.75, -15.83) radius 1.5
  circle A40 centre (-90.25, -15.83) radius 1.5
  circle A41 centre (-97.75, -15.83) radius 1.5
  circle A42 centre (-105.25, -15.83) radius 1.5
  circle A43 centre (-82.75, -3.83) radius 1.5
  circle A44 centre (-90.25, -3.83) radius 1.5
  circle A45 centre (-97.75, -3.83) radius 1.5
  circle A46 centre (-105.25, -3.83) radius 1.5
  circle A47 centre (-82.75, 8.17) radius 1.5
  circle A48 centre (-90.25, 8.17) radius 1.5
  circle A49 centre (-97.75, 8.17) radius 1.5
  circle A50 centre (-105.25, 8.17) radius 1.5
  circle A51 centre (-82.75, 20.17) radius 1.5
  circle A52 centre (-90.25, 20.17) radius 1.5
  circle A53 centre (-97.75, 20.17) radius 1.5
  circle A54 centre (-105.25, 20.17) radius 1.5
  circle A55 centre (-82.75, 32.17) radius 1.5
  circle A56 centre (-90.25, 32.17) radius 1.5
  circle A57 centre (-97.75, 32.17) radius 1.5
  circle A58 centre (-105.25, 32.17) radius 1.5
  circle A59 centre (-31.75, 6.0325) radius 1.5
  circle A60 centre (-31.75, -18.0975) radius 1.5
  circle A61 centre (-6.35, -18.0975) radius 1.5
  circle A62 centre (-6.35, 18.0975) radius 1.5
  circle A63 centre (19.05, 18.0975) radius 1.5
  circle A64 centre (6.35, -18.0975) radius 1.5
  circle A65 centre (31.75, 6.0325) radius 1.5
  circle A66 centre (44.45, -6.0325) radius 1.5
  circle A67 centre (38.1, 24.13) radius 1.5
  circle A68 centre (0, 24.13) radius 1.5
  circle A69 centre (-25.4, -24.13) radius 1.5
  circle A70 centre (-12.7, -24.13) radius 1.5
  circle A71 centre (12.7, 12.065) radius 1.5
  circle A72 centre (50.8, -24.13) radius 1.5
  circle A73 centre (-50.8, -24.13) radius 1.5
  circle A74 centre (12.7, -12.065) radius 1.5
  circle A75 centre (-25.4, -12.065) radius 1.5
  circle A76 centre (50.8, 12.065) radius 1.5
  circle A77 centre (-38.1, 0) radius 1.5
  circle A78 centre (-50.8, 24.13) radius 1.5
  circle A79 centre (-12.7, -12.065) radius 1.5
  circle A80 centre (-38.1, -12.065) radius 1.5
  circle A81 centre (-38.1, -24.13) radius 1.5
  circle A82 centre (25.4, 0) radius 1.5
  circle A83 centre (25.4, -24.13) radius 1.5
  circle A84 centre (12.7, -24.13) radius 1.5
  circle A85 centre (38.1, -12.065) radius 1.5
  circle A86 centre (-38.1, 24.13) radius 1.5
  circle A87 centre (0, 12.065) radius 1.5
  circle A88 centre (-25.4, 0) radius 1.5
  circle A89 centre (44.45, -18.0975) radius 1.5
  circle A90 centre (31.75, 18.0975) radius 1.5
  circle A91 centre (19.05, -18.0975) radius 1.5
  circle A92 centre (19.05, 6.0325) radius 1.5
  circle A93 centre (-6.35, 6.0325) radius 1.5
  circle A94 centre (-6.35, -6.0325) radius 1.5
  circle A95 centre (-31.75, -6.0325) radius 1.5
  circle A96 centre (-44.45, 6.0325) radius 1.5
  circle A97 centre (-31.75, 18.0975) radius 1.5
  circle A98 centre (-44.45, -18.0975) radius 1.5
  circle A99 centre (-19.05, -18.0975) radius 1.5
  circle A100 centre (-19.05, 18.0975) radius 1.5
  circle A101 centre (6.35, 18.0975) radius 1.5
  circle A102 centre (6.35, -6.0325) radius 1.5
  circle A103 centre (31.75, -6.0325) radius 1.5
  circle A104 centre (44.45, 6.0325) radius 1.5
  circle A105 centre (25.4, 24.13) radius 1.5
  circle A106 centre (38.1, 0) radius 1.5
  circle A107 centre (-50.8, -12.065) radius 1.5
  circle A108 centre (-25.4, 24.13) radius 1.5
  circle A109 centre (-38.1, 12.065) radius 1.5
  circle A110 centre (38.1, -24.13) radius 1.5
  circle A111 centre (-50.8, 0) radius 1.5
  circle A112 centre (50.8, -12.065) radius 1.5
  circle A113 centre (38.1, 12.065) radius 1.5
  circle A114 centre (-50.8, 12.065) radius 1.5
  circle A115 centre (0, -24.13) radius 1.5
  circle A116 centre (-12.7, 0) radius 1.5
  circle A117 centre (12.7, 24.13) radius 1.5
  circle A118 centre (25.4, 12.065) radius 1.5
  circle A119 centre (-25.4, 12.065) radius 1.5
  circle A120 centre (12.7, 0) radius 1.5
  circle A121 centre (-12.7, 24.13) radius 1.5
  circle A122 centre (25.4, -12.065) radius 1.5
  circle A123 centre (0, 0) radius 1.5
  circle A124 centre (50.8, 0) radius 1.5
  circle A125 centre (50.8, 24.13) radius 1.5
  circle A126 centre (0, -12.065) radius 1.5
  circle A127 centre (-12.7, 12.065) radius 1.5
  circle A128 centre (44.45, 18.0975) radius 1.5
  circle A129 centre (31.75, -18.0975) radius 1.5
  circle A130 centre (19.05, -6.0325) radius 1.5
  circle A131 centre (6.35, 6.0325) radius 1.5
  circle A132 centre (-19.05, 6.0325) radius 1.5
  circle A133 centre (-19.05, -6.0325) radius 1.5
  circle A134 centre (-44.45, -6.0325) radius 1.5
  circle A135 centre (-44.45, 18.0975) radius 1.5
  circle A136 centre (58.42, -31.75) radius 3.9
  circle A137 centre (58.42, 31.75) radius 3.9
  line L12 (67.5, 39.83) -> (-11.62, 39.83)
  line L13 (-11.62, 39.83) -> (-11.62, 44.17)
  line L14 (67.5, -39.83) -> (67.5, 39.83)
  circle A138 centre (-58.42, 31.75) radius 3.9
  circle A139 centre (-58.42, -31.75) radius 3.9
  line L15 (-67.5, 44.17) -> (-67.5, -22.83)
  line L16 (-67.5, -22.83) -> (-72.5, -22.83)
  line L17 (-72.5, -22.83) -> (-72.5, 44.17)
  line L18 (-72.5, 44.17) -> (-115.5, 44.17)
  line L19 (-94, 44.17) -> (-94, -39.83) construction
  line L20 (-72.5, 44.17) -> (-72.5, -39.83) construction
  dimension "d176" = 3
  dimension "d179" = 15
  dimension "d180" = 36
  dimension "d181" = 3
  dimension "d184" = -22.5
  dimension "d185" = 60
  constraint coincident L1 L5.end
  constraint perpendicular L1 L5
  constraint coincident A5.centre L6.start
  constraint coincident A10.centre L6.end
  constraint coincident A9.centre L7.end
  constraint coincident A4.centre L8.end
  constraint midpoint L6 L10.start
  constraint midpoint L8 L10.end
  constraint midpoint L9 L11.start
  constraint midpoint L7 L11.end
  constraint midpoint L10 A35.centre
  constraint midpoint L18 L19.start
  constraint coincident L4 L19.end
  constraint vertical L19
  constraint coincident L5 A0.centre
  constraint coincident A0.centre L19
  constraint coincident L17.end L18.start
  constraint coincident L4 L20.end
  constraint perpendicular L4 L20
  constraint midpoint L5.start L20
  measures "d176" diameter of A0
  measures "d181" diameter of A35
extrude "Extrude22" cut sketch "Sketch19" against normal up to surface (5 mm away) contours A0 | A1 | A2 | A3 | A4 | A5 | A6 | A7 | A8 | A9 | A10 | A11 | A12 | A13 | A14 | A15 | A16 | A17 | A18 | A19 | A20 | A21 | A22 | A23 | A24 | A25 | A26 | A27 | A28 | A29 | A30 | A31 | A32 | A33 | A34 | A35 | A36 | A37 | A38 | A39 | A40 | A41 | A42 | A43 | A44 | A45 | A46 | A47 | A48 | A49 | A50 | A51 | A52 | A53 | A54 | A55 | A56 | A57 | A58 bodies 1
fillet "Fillet2" [suppressed]
equation "d1 = 5 in + 8 mm"
equation "d2 = d1 / 2"
equation "d3 = 2.9 in + 6 mm"
equation "d4 = d3 / 2"
equation "d9 = d1 / 2 - 0.2 in - 4 mm"
equation "d10 = d9"
equation "d11 = d9"
equation "d12 = d9"
equation "d13 = d3 / 2 - 0.2 in - 3 mm"
equation "d14 = d13"
equation "d15 = d13"
equation "d16 = d13"
equation "d18 = d17"
equation "d19 = d17"
equation "d20 = d18"
equation "d21 = d17 + 4 mm"
equation "d22 = d21"
equation "d23 = d21"
equation "d24 = d21"
equation "d25 = 5 mm"
equation "d29 = d25 + 30 mm"
equation "d39 = d33 / 2"
equation "d40 = d39"
equation "d42 = d39"
equation "d43 = d121"
equation "d44 = d41"
equation "d46 = d39"
equation "d47 = d41"
equation "d48 = d39"
equation "d50 = d41"
equation "d60 = 2.8 in + 8 mm"
equation "d63 = 1.65 in + 8 mm - d29"
equation "d66 = d65"
equation "d67 = d65"
equation "d69 = -d59 + 3 mm"
equation "d80 = d79"
equation "d81 = d79"
equation "d82 = d79"
equation "d85 = 0.2 in + 1 mm"
equation "d86 = d85"
equation "d87 = d85"
equation "d88 = d85"
equation "d89 = d85"
equation "d91 = d85"
equation "d113 = d5"
equation "d114 = d8"
equation "d115 = d8"
equation "d116 = d33"
equation "d122 = d39"
equation "d131 = d85"
equation "d132 = d85"
equation "d133 = d79 + 3 mm"
equation "d134 = d133"
equation "d135 = d133"
equation "d136 = d133"
equation "d140 = d65"
equation "d171 = d168"
equation "d181 = d176"
